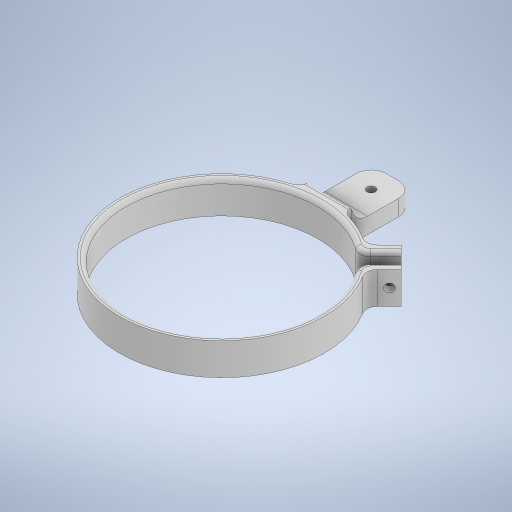
# Autodesk Inventor part: HopperMount
Saved by Autodesk Inventor 2024.2 (Build 282272000, 272)
## iProperties
Created: 2024-06-03
Part Number: HopperMount
Material: Generic
Document SubType Name: Modeling
Designer: Robin
Density: 1 g/cm^3
Appearance: Default
Author: Robin
Autodesk Inventor part; units mm, degrees
ref_plane "YZ Plane" through (0, 0, 0) normal (1, 0, 0) x (0, 1, 0)
ref_plane "XZ Plane" through (0, 0, 0) normal (0, 1, 0) x (-1, 0, 0)
ref_plane "XY Plane" through (0, 0, 0) normal (0, 0, 1) x (1, 0, 0)
sketch "Sketch1" plane through (0, 0, 0) normal (0, 1, 0) x (-1, 0, 0)
  circle A0 centre (0, 0) radius 48
  circle A1 centre (0, 0) radius 45
  line L0 (10, -45) -> (-10, -45)
  line L1 (-10, -45) -> (-10, -80)
  line L2 (-10, -80) -> (10, -80)
  line L3 (10, -80) -> (10, -45)
  line L4 (-4, 44.8219) -> (4, 44.8219)
  circle A2 centre (0, -70) radius 10
  circle A3 centre (0, -70) radius 2
  line L5 (0, 0) -> (-57.7849, -57.7849)
  line L6 (0, 0) -> (0, -45)
  line L7 (-26.4827, -36.3822) -> (-36.3822, -26.4827)
  line L8 (-36.3822, -26.4827) -> (-46.9888, -37.0893)
  line L9 (-46.9888, -37.0893) -> (-37.0893, -46.9888)
  line L10 (-37.0893, -46.9888) -> (-26.4827, -36.3822)
  line L11 (-29.3111, -33.5538) -> (-33.5538, -29.3111)
  line L12 (-33.5538, -29.3111) -> (-44.1604, -39.9177)
  line L13 (-44.1604, -39.9177) -> (-39.9177, -44.1604)
  line L14 (-39.9177, -44.1604) -> (-29.3111, -33.5538)
  point P0 (0, 45)
  point P1 (4, 60)
  point P2 (-10, -46.9468)
  point P3 (10, -46.9468)
  point P4 (10, -70)
  point P5 (-10, -70)
  point P6 (0, -45)
  point P7 (0, -80)
  point P8 (-28.6285, -38.528)
  point P9 (-38.528, -28.6285)
  point P10 (-29.6277, -33.8703)
  point P11 (-33.8703, -29.6277)
  dimension "d0" = 96
  dimension "d1" = 90
  dimension "d2" = 20
  dimension "d13" = 35
  dimension "d14" = 4
  dimension "d15" = 45
  dimension "d16" = 7
  dimension "d17" = 7
  dimension "d18" = 15
  dimension "d19" = 3
  dimension "d20" = 3
  constraints: 30 end point, 6 perpendicular, 4 centre point, 4 parallel, 4 point on circle, 4 tangent, 3 coincident, 2 collinear, 2 vertical alignment, 1 horizontal, 1 midpoint, 1 point on line, 1 vertical
  measures "d0" diameter of A0
  measures "d1" diameter of A1
  measures "d2" distance of L1.end L2.end
  measures "d13" distance of L2.end L0.start
  measures "d14" diameter of A3
  measures "d15" angle of L6 L5
  measures "d16" distance between parallel lines of L8 L5
  measures "d17" distance between parallel lines of L5 L10
  measures "d18" distance of L7.end L8.end
  measures "d19" distance between parallel lines of L5 L12
  measures "d20" distance between parallel lines of L5 L14
extrude "Extrusion1" add sketch "Sketch1" along normal blind 15 contours A0 L3 L0 A1 L8 | L8 A1 L12 A0 | A0 L12 L9 L8 | L3 A2 L1 A0 | A0 L1 L0 L3 | A0 L10 A1 L0 L1 | A2 | L3 L2 A2 | L10 L9 L14 A0 | A0 L14 A1 L10 | A2 L2 L1
fillet "Fillet1" radius 5 6 edges at (38.528, 7.5, -28.6285) (28.6285, 7.5, -38.528) (10, 7.5, -46.9468) (-10, 7.5, -46.9468) (33.8703, 7.5, -29.6277) (29.6277, 7.5, -33.8703)
sketch "Sketch5" plane through (10, 0, -80) normal (1, 0, 0) x (0, 0, -1)
  line L0 (0, 15) -> (-29.1669, 15) projected
  line L1 (0, 0) -> (0, 15) projected
  line L2 (-29.1669, 15) -> (0, 15)
  line L3 (0, 15) -> (0, 7.5)
  line L4 (0, 7.5) -> (-29.1669, 7.5)
  line L5 (-29.1669, 7.5) -> (-29.1669, 15)
  arc A0 (-29.1669, 15) -> (-21.6669, 7.5) centre (-21.6669, 15) ccw
  line L6 (-29.1669, 0) -> (-29.1669, 15) projected
  point P0 (-80, 0)
  constraints: 8 end point, 2 parallel, 2 point on circle, 2 tangent, 1 centre point, 1 horizontal, 1 midpoint, 1 perpendicular, 1 point on line
extrude "Extrusion3" cut sketch "Sketch5" against normal through all contours L1 L4 A0 L0
fillet "Fillet2" radius 7 2 edges at (10, 3.75, -80) (-10, 3.75, -80)
sketch "Sketch6" plane through (46.9888, 0, -37.0893) normal (0.7071, 0, 0.7071) x (0.7071, 0, -0.7071)
  circle A0 centre (-3.9143, 7.5) radius 2
  line L0 (0, 0) -> (0, 15) projected
  line L1 (-7.8286, 15) -> (0, 15) projected
  point P0 (-59.4522, 0)
  point P1 (0, 7.5)
  point P2 (-3.9143, 15)
  dimension "d25" = 4
  constraints: 2 midpoint, 1 centre point, 1 horizontal alignment, 1 vertical alignment
  measures "d25" diameter of A0
extrude "Extrusion4" cut sketch "Sketch6" against normal up to surface (14 mm away)
fillet "Fillet3" radius 2 1 edges at (0, 15, -50.8331)
fillet "Fillet4" radius 2 5 edges at (-31.8198, 15, 31.8198) (29.6443, 15, -35.5728) (36.3481, 15, -40.5908) (35.5728, 15, -29.6443) (40.5908, 15, -36.3481)
body "Solid1"
